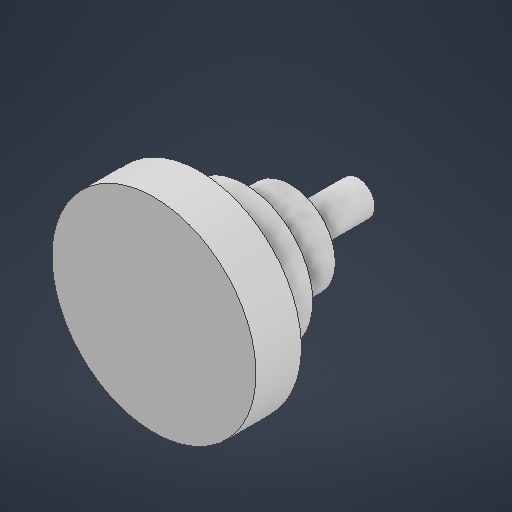
# Autodesk Inventor part: Part2
Saved by Autodesk Inventor 2026 (Build 300175050, 175E)
## iProperties
Created: 2026-03-26
Part Number: Part2
Material: Generic
Document SubType Name: Modeling
Designer: Administrator
Density: 1 g/cm^3
Appearance: Default
Author: Administrator
Autodesk Inventor part; units mm, degrees
ref_plane "YZ Plane" through (0, 0, 0) normal (1, 0, 0) x (0, 1, 0)
ref_plane "XZ Plane" through (0, 0, 0) normal (0, 1, 0) x (-1, 0, 0)
ref_plane "XY Plane" through (0, 0, 0) normal (0, 0, 1) x (1, 0, 0)
sketch "Sketch1" plane through (0, 0, 0) normal (1, 0, 0) x (0, 1, 0)
  line L0 (0, 0) -> (0, -90)
  line L1 (0, -90) -> (7.5, -90)
  line L2 (7.5, -90) -> (7.5, -60)
  line L3 (7.5, -60) -> (20, -60)
  line L4 (20, -60) -> (20, -40)
  line L5 (20, -40) -> (30, -40)
  line L6 (30, -40) -> (30, -20)
  line L7 (30, -20) -> (45, -20)
  line L8 (45, -20) -> (45, 0)
  line L9 (45, 0) -> (0, 0)
  dimension "d0" = 90
  dimension "d1" = 15
  dimension "d2" = 40
  dimension "d3" = 60
  dimension "d4" = 90
  dimension "d5" = 20
  dimension "d6" = 20
  dimension "d7" = 20
  constraints: 20 end point, 8 perpendicular, 1 horizontal, 1 vertical
  measures "d0" distance of L0.start L0.end
  measures "d1" diameter of L2 L0
  measures "d2" diameter of L4 L0
  measures "d3" diameter of L6 L0
  measures "d4" diameter of L8 L0
  measures "d5" distance of L7.end L8.end
  measures "d6" distance of L5.end L6.end
  measures "d7" distance of L3.end L4.end
revolve "Revolution1" add sketch "Sketch1" angle 360 about axis through (0, 0, 0) along (0, 0, -1)
body "Solid1"
